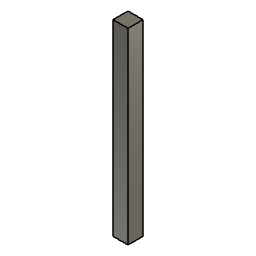
뎁스 기준점 (Autodesk Fusion 360 design; units mm, degrees)
Autodesk Fusion 360 part; units mm, degrees
sketch "스케치1" plane through (0, 0, 0) normal (0, 0, 1) x (1, 0, 0)
  line L0 (1.5, 1.5) -> (-1.5, 1.5)
  line L1 (-1.5, 1.5) -> (-1.5, -1.5)
  line L2 (-1.5, -1.5) -> (1.5, -1.5)
  line L3 (1.5, -1.5) -> (1.5, 1.5)
  line L4 (1.5, 1.5) -> (-1.5, -1.5) construction
  line L5 (-1.5, 1.5) -> (1.5, -1.5) construction
  dimension "d1" = 3
  dimension "d2" = 3
  constraint horizontal L0
  constraint perpendicular L0 L1
  constraint parallel L0 L2
  constraint parallel L1 L3
  constraint coincident L4 origin
  constraint coincident L5 origin
  measures "d1" distance of L1.end L2.end
  measures "d2" distance of L0.end L1.end
extrude "돌출1" add sketch "스케치1" along normal blind 37.5
